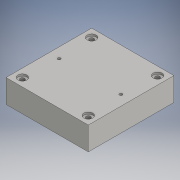
# Autodesk Inventor part: NUCBasePCB
Saved by Autodesk Inventor 2016 (Build 200138000, 138)
## iProperties
Created: 2015-09-23
Part Number: NUCBasePCB
Material: Generic
Document SubType Name: Modeling
Designer: lachesis
Density: 1 g/cm^3
Appearance: Default
Author: lachesis
Autodesk Inventor part; units mm, degrees
ref_plane "YZ Plane" through (0, 0, 0) normal (1, 0, 0) x (0, 1, 0)
ref_plane "XZ Plane" through (0, 0, 0) normal (0, 1, 0) x (-1, 0, 0)
ref_plane "XY Plane" through (0, 0, 0) normal (0, 0, 1) x (1, 0, 0)
sketch "Sketch1" plane through (0, 0, 0) normal (0, 1, 0) x (-1, 0, 0)
  line L0 (58.42, 56.134) -> (-58.42, 56.134)
  line L1 (-58.42, 56.134) -> (-58.42, -56.134)
  line L2 (-58.42, -56.134) -> (58.42, -56.134)
  line L3 (58.42, -56.134) -> (58.42, 56.134)
  point P0 (0, 0)
  point P1 (0, -56.134)
  point P2 (58.42, 0)
  dimension "d0" = 112.268
  dimension "d1" = 116.84
  constraints: 8 end point, 2 midpoint, 2 parallel, 1 horizontal, 1 horizontal alignment, 1 perpendicular, 1 vertical alignment
  measures "d0" distance of L2.end L0.start
  measures "d1" distance of L1.end L2.end
extrude "Extrusion1" add sketch "Sketch1" along normal blind 31.75
sketch "Sketch2" plane through (0, 31.75, 0) normal (0, 1, 0) x (1, 0, 0)
  line L0 (58.42, -56.134) -> (58.42, 56.134) projected
  line L1 (58.42, 56.134) -> (-58.42, 56.134) projected
  line L2 (-58.42, -56.134) -> (58.42, -56.134) projected
  line L3 (-58.42, 56.134) -> (-58.42, -56.134) projected
  point P0 (0, 0)
  point P1 (47.244, 44.958)
  point P2 (47.244, -44.958)
  point P3 (-47.244, 44.958)
  point P4 (-47.244, -44.958)
  dimension "d4" = 11.176
  dimension "d5" = 11.176
  dimension "d6" = 11.176
  dimension "d7" = 11.176
  constraints: 2 horizontal alignment, 2 vertical alignment
  measures "d4" distance from line of L0 point (47.244, 44.958)
  measures "d5" distance from line of L1 point (47.244, 44.958)
  measures "d6" distance from line of L2 point (-47.244, -44.958)
  measures "d7" distance from line of L3 point (-47.244, -44.958)
hole "Hole1" at (47.244, 31.75, -44.958) at (47.244, 31.75, 44.958) at (-47.244, 31.75, -44.958) at (-47.244, 31.75, 44.958) direction (0, -1, 0) diameter 3.302 end through all counterbore diameter 5.969 counterbore depth 26.162
sketch "Sketch3" plane through (0, 31.75, 0) normal (0, 1, 0) x (1, 0, 0)
  circle A0 centre (47.244, 44.958) radius 2.9845 projected
  circle A1 centre (47.244, -44.958) radius 2.9845 projected
  circle A2 centre (-47.244, 44.958) radius 2.9845 projected
  circle A3 centre (-47.244, -44.958) radius 2.9845 projected
  circle A4 centre (47.244, 44.958) radius 1.651 projected
  circle A5 centre (47.244, -44.958) radius 1.651 projected
  circle A6 centre (-47.244, -44.958) radius 1.651 projected
  point P0 (0, 0)
  constraints: 4 coincident
hole "Hole2" at (47.244, 31.75, -44.958) at (47.244, 31.75, 44.958) at (-47.244, 31.75, 44.958) at (-47.244, 31.75, -44.958) direction (0, -1, 0) diameter 12.065 depth 2.413
sketch "Sketch5" plane through (0, 0, 0) normal (0, -1, 0) x (1, 0, 0)
  circle A0 centre (-47.244, 44.958) radius 1.651 projected
  circle A1 centre (-47.244, -44.958) radius 1.651 projected
  point P0 (0, 0)
  point P1 (0, 42.164)
  point P2 (0, -42.164)
  dimension "d25" = 47.244
  dimension "d26" = 2.794
  dimension "d27" = 2.794
  constraints: 1 vertical alignment
  measures "d25" horizontal distance of A0.centre point (0, 42.164)
  measures "d26" vertical distance of A0.centre point (0, 42.164)
  measures "d27" vertical distance of A1.centre point (0, -42.164)
hole "Hole3" at (0, 0, 42.164) at (0, 0, -42.164) direction (0, 1, 0) diameter 3.9116 end through all counterbore diameter 6.604 counterbore depth 19.558
equation "\"d5\" = d4"
equation "\"d6\" = d4"
equation "\"d7\" = d4"
body "Solid1"
